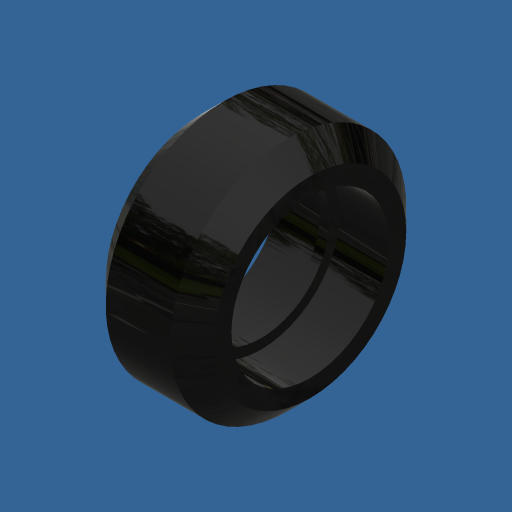
# Autodesk Inventor part: V-Slot wheel
Saved by Autodesk Inventor 2023 (Build 270158030, 158C)
## iProperties
Created: 2023-02-04
Part Number: V-Slot wheel
Material: Acetal Resin, Black
Document SubType Name: Modeling
Designer: kumpu
Density: 1.425 g/cm^3
Appearance: Smooth - Black
Author: kumpu
Autodesk Inventor part; units mm, degrees
ref_plane "YZ Plane" through (0, 0, 0) normal (1, 0, 0) x (0, 1, 0)
ref_plane "XZ Plane" through (0, 0, 0) normal (0, 1, 0) x (-1, 0, 0)
ref_plane "XY Plane" through (0, 0, 0) normal (0, 0, 1) x (1, 0, 0)
sketch "Sketch1" plane through (0, 0, 0) normal (0, 0, 1) x (1, 0, 0)
  line L0 (-5.5, 9.77) -> (-5.5, 8)
  line L1 (-5.5, 8) -> (-0.5, 8)
  line L2 (-0.5, 8) -> (-0.5, 7)
  line L3 (-0.5, 7) -> (0.5, 7)
  line L4 (0.5, 7) -> (0.5, 8)
  line L5 (0.5, 8) -> (5.5, 8)
  line L6 (5.5, 8) -> (5.5, 9.77)
  line L7 (5.5, 9.77) -> (3.27, 12)
  line L8 (3.27, 12) -> (-3.27, 12)
  line L9 (-3.27, 12) -> (-5.5, 9.77)
  line L10 (0, 7) -> (0, 0) construction
  line L11 (0, 0) -> (-5.5, 0) construction
  dimension "d0" = 11
  dimension "d1" = 16
  dimension "d2" = 9.77
  dimension "d3" = 24
  dimension "d4" = 1
  dimension "d5" = 1
  constraints: 24 end point, 6 perpendicular, 3 equal length, 3 point on line, 2 vertical, 1 horizontal, 1 midpoint, 1 parallel
  measures "d0" distance between parallel lines of L6 L0
  measures "d1" diameter of L1 L11
  measures "d2" distance of L11.end L0.start
  measures "d3" diameter of L8 L11
  measures "d4" distance of L2.end L3.end
  measures "d5" distance of L1.end L2.end
revolve "Revolution1" add sketch "Sketch1" angle 360 about axis through (0, 0, 0) along (-1, 0, 0)
body "Solid1"
